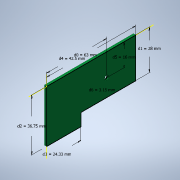
# Autodesk Inventor part: J010361
Saved by Autodesk Inventor 2020.3 (Build 243373000, 373)
## iProperties
RuleStatus: InUse
AfterDocSave0: file://Part Number Cleaner
Created: 2022-05-31
Part Number: J010361
Material: FR4
Catalog Web Link: https://www.janelia.org/
Vendor: HHMI: JRC - jET
Document SubType Name: Modeling
Designer: arnoldj
Density: 1.1 g/cm^3
Appearance: Green (Flat)
Project: COMMON
Description: RGB DOUT PCB
LAB/DEPT: COMMON
REQUESTING SCIENTIST: COMMON
SURFACE ROUGHNESS: N/A
DESIGN DEPARTMENT: HHMI: JRC - jET
SPECIAL FINISH: NONE
ALTERED ITEM PART NUMBER: N/A
ALTERED ITEM VENDOR: N/A
ALTERED ITEM DESCRIPTION: N/A
Title: Standard
Author: arnoldj
Revision Number: 0
Autodesk Inventor part; units mm, degrees
ref_plane "YZ Plane" through (0, 0, 0) normal (1, 0, 0) x (0, 1, 0)
ref_plane "XZ Plane" through (0, 0, 0) normal (0, 1, 0) x (-1, 0, 0)
ref_plane "XY Plane" through (0, 0, 0) normal (0, 0, 1) x (1, 0, 0)
sketch "Sketch1" plane through (0, 0, 0) normal (1, 0, 0) x (0, 1, 0)
  line L0 (0, 12.6) -> (0, -75.6) projected
  line L1 (-44.1, 0) -> (7.35, 0) projected
  line L2 (0, 0) -> (0, -63)
  line L3 (0, -63) -> (-28, -63)
  line L4 (-28, -63) -> (-28, -24.33)
  line L5 (-28, -24.33) -> (-36.75, -24.33)
  line L6 (-36.75, -24.33) -> (-36.75, 0)
  line L7 (-36.75, 0) -> (0, 0)
  circle A0 centre (-16, -42.5) radius 1.575 construction
  dimension "d0" = 63
  dimension "d1" = 28
  dimension "d2" = 36.75
  dimension "d3" = 24.33
  dimension "d4" = 42.5
  dimension "d5" = 16
  dimension "d6" = 3.15
  constraints: 12 end point, 3 perpendicular, 2 horizontal, 2 point on line, 1 centre point, 1 coincident
  measures "d0" distance between parallel lines of L1 L3
  measures "d1" distance of L2.end L3.end
  measures "d2" distance between parallel lines of L6 L2
  measures "d3" distance of L5.end L6.end
  measures "d4" distance from line of L7 point (-16, -42.5)
  measures "d5" distance from line of point (-16, -42.5) L2
  measures "d6" diameter of A0
extrude "Extrusion1" add sketch "Sketch1" against normal blind 1.55
hole "Hole1" at (0, -16, -42.5) direction (-1, 0, 0) diameter 3.15 end through all
body "Solid1"
